Autodesk Inventor part; units mm, degrees
(part 5 of 5)
sketch "Эскиз12" plane through (0, 2, 0) normal (0, 1, 0) x (1, 0, 0)
  line L0 (-0.8, -32.5335) -> (0.8, -32.5335)
  line L1 (0.8, -32.5335) -> (0.8, -39.5335)
  line L2 (0.8, -39.5335) -> (-0.8, -39.5335)
  line L3 (-0.8, -39.5335) -> (-0.8, -32.5335)
  line L4 (-0.8, -32.5335) -> (0.8, -39.5335) construction
  line L5 (35.896, -32.6933) -> (41.3657, -27.2236) construction
  arc A0 (44.1942, -27.2236) -> (41.3657, -27.2236) centre (42.78, -28.6378) ccw construction
  line L6 (44.1942, -27.2236) -> (63.6396, -46.669) construction
  line L7 (63.6396, -46.669) -> (46.669, -63.6396) construction
  line L8 (46.669, -63.6396) -> (27.2236, -44.1942) construction
  arc A1 (27.2236, -41.3657) -> (27.2236, -44.1942) centre (28.6378, -42.78) ccw construction
  line L9 (27.2236, -41.3657) -> (31.4801, -37.1092) construction
  arc A2 (31.4801, -37.1092) -> (35.896, -32.6933) centre (31.9203, -33.1335) ccw construction
  circle A3 centre (0, -54) radius 1.6 construction
  arc A4 (-93.0503, 48.6481) -> (-93.0503, -48.6481) centre (0, 0) ccw construction
  arc A5 (-93.0503, -48.6481) -> (-88.2704, -49.3795) centre (-90.3917, -47.2582) ccw construction
  line L10 (-88.2704, -49.3795) -> (-85.2064, -46.3155) construction
  arc A6 (-73.8927, -46.3155) -> (-85.2064, -46.3155) centre (-79.5495, -51.9723) ccw construction
  line L11 (-73.8927, -46.3155) -> (-46.3155, -73.8927) construction
  arc A7 (-46.3155, -85.2064) -> (-46.3155, -73.8927) centre (-51.9723, -79.5495) ccw construction
  line L12 (-46.3155, -85.2064) -> (-49.3795, -88.2704) construction
  arc A8 (-49.3795, -88.2704) -> (-48.6481, -93.0503) centre (-47.2582, -90.3917) ccw construction
  arc A9 (-48.6481, -93.0503) -> (-45.42, -94.668) centre (0, 0) ccw construction
  arc A10 (-45.42, -94.668) -> (-43.0355, -94.1655) centre (-44.5548, -92.8648) ccw construction
  line L13 (-43.0355, -94.1655) -> (-18.3802, -65.3664) construction
  arc A11 (-17.477, -64.7643) -> (-18.3802, -65.3664) centre (-16.8609, -66.6671) ccw construction
  line L14 (-17.477, -64.7643) -> (-0.6161, -59.3045) construction
  arc A12 (0.6161, -59.3045) -> (-0.6161, -59.3045) centre (0, -61.2072) ccw construction
  line L15 (0.6161, -59.3045) -> (17.477, -64.7643) construction
  arc A13 (18.3802, -65.3664) -> (17.477, -64.7643) centre (16.8609, -66.6671) ccw construction
  line L16 (18.3802, -65.3664) -> (43.0355, -94.1655) construction
  arc A14 (43.0355, -94.1655) -> (45.42, -94.668) centre (44.5548, -92.8648) ccw construction
  arc A15 (45.42, -94.668) -> (48.6481, -93.0503) centre (0, 0) ccw construction
  arc A16 (48.6481, -93.0503) -> (49.3795, -88.2704) centre (47.2582, -90.3917) ccw construction
  line L17 (49.3795, -88.2704) -> (46.3155, -85.2064) construction
  arc A17 (46.3155, -73.8927) -> (46.3155, -85.2064) centre (51.9723, -79.5495) ccw construction
  line L18 (46.3155, -73.8927) -> (73.8927, -46.3155) construction
  arc A18 (85.2064, -46.3155) -> (73.8927, -46.3155) centre (79.5495, -51.9723) ccw construction
  line L19 (85.2064, -46.3155) -> (88.2704, -49.3795) construction
  arc A19 (88.2704, -49.3795) -> (93.0503, -48.6481) centre (90.3917, -47.2582) ccw construction
  arc A20 (93.0503, -48.6481) -> (93.0503, 48.6481) centre (0, 0) ccw construction
  arc A21 (93.0503, 48.6481) -> (88.2704, 49.3795) centre (90.3917, 47.2582) ccw construction
  line L20 (88.2704, 49.3795) -> (85.2064, 46.3155) construction
  arc A22 (73.8927, 46.3155) -> (85.2064, 46.3155) centre (79.5495, 51.9723) ccw construction
  line L21 (73.8927, 46.3155) -> (46.3155, 73.8927) construction
  arc A23 (46.3155, 85.2064) -> (46.3155, 73.8927) centre (51.9723, 79.5495) ccw construction
  line L22 (46.3155, 85.2064) -> (49.3795, 88.2704) construction
  arc A24 (49.3795, 88.2704) -> (48.6481, 93.0503) centre (47.2582, 90.3917) ccw construction
  arc A25 (48.6481, 93.0503) -> (11.8382, 104.3305) centre (0, 0) ccw construction
  arc A26 (11.8382, 104.3305) -> (8.5, 101.3496) centre (11.5, 101.3496) ccw construction
  line L23 (8.5, 101.3496) -> (8.5, 90.5) construction
  arc A27 (7, 89) -> (8.5, 90.5) centre (7, 90.5) ccw construction
  line L24 (7, 89) -> (-7, 89) construction
  arc A28 (-8.5, 90.5) -> (-7, 89) centre (-7, 90.5) ccw construction
  line L25 (-8.5, 90.5) -> (-8.5, 101.3496) construction
  arc A29 (-8.5, 101.3496) -> (-11.8382, 104.3305) centre (-11.5, 101.3496) ccw construction
  arc A30 (-11.8382, 104.3305) -> (-48.6481, 93.0503) centre (0, 0) ccw construction
  arc A31 (-48.6481, 93.0503) -> (-49.3795, 88.2704) centre (-47.2582, 90.3917) ccw construction
  line L26 (-49.3795, 88.2704) -> (-46.3155, 85.2064) construction
  arc A32 (-46.3155, 73.8927) -> (-46.3155, 85.2064) centre (-51.9723, 79.5495) ccw construction
  line L27 (-46.3155, 73.8927) -> (-73.8927, 46.3155) construction
  arc A33 (-85.2064, 46.3155) -> (-73.8927, 46.3155) centre (-79.5495, 51.9723) ccw construction
  line L28 (-85.2064, 46.3155) -> (-88.2704, 49.3795) construction
  arc A34 (-88.2704, 49.3795) -> (-93.0503, 48.6481) centre (-90.3917, 47.2582) ccw construction
  arc A35 (-90.4395, 37.7453) -> (-97.9653, 2.6059) centre (0, 0) ccw construction
  arc A36 (-87.1795, 38.3892) -> (-90.4395, 37.7453) centre (-88.5938, 36.975) ccw construction
  line L29 (-87.1795, 38.3892) -> (-83.085, 34.2947) construction
  arc A37 (-83.085, 34.2947) -> (-76.014, 34.2947) centre (-79.5495, 37.8302) ccw construction
  line L30 (-76.014, 34.2947) -> (-67.8823, 42.4264) construction
  line L31 (-67.8823, 42.4264) -> (-47.1257, 21.6698) construction
  arc A38 (-47.1257, 21.6698) -> (-43.384, 17.9282) centre (-43.1335, 21.9203) ccw construction
  line L32 (-43.384, 17.9282) -> (-26.8701, 1.4142) construction
  arc A39 (-26.8701, -1.4142) -> (-26.8701, 1.4142) centre (-28.2843, 0) ccw construction
  line L33 (-26.8701, -1.4142) -> (-43.384, -17.9282) construction
  arc A40 (-43.384, -17.9282) -> (-47.1257, -21.6698) centre (-43.1335, -21.9203) ccw construction
  line L34 (-47.1257, -21.6698) -> (-67.8823, -42.4264) construction
  line L35 (-67.8823, -42.4264) -> (-76.014, -34.2947) construction
  arc A41 (-76.014, -34.2947) -> (-83.085, -34.2947) centre (-79.5495, -37.8302) ccw construction
  line L36 (-83.085, -34.2947) -> (-87.1795, -38.3892) construction
  arc A42 (-90.4395, -37.7453) -> (-87.1795, -38.3892) centre (-88.5938, -36.975) ccw construction
  arc A43 (-97.9653, -2.6059) -> (-90.4395, -37.7453) centre (0, 0) ccw construction
  arc A44 (-97.9653, -2.6059) -> (-97.9653, 2.6059) centre (-101, 0) ccw construction
  line L37 (29.746, -55.2019) -> (42.4264, -67.8823) construction
  line L38 (42.4264, -67.8823) -> (37.1244, -73.1843) construction
  arc A45 (34.1909, -73.0707) -> (37.1244, -73.1843) centre (35.7102, -71.7701) ccw construction
  line L39 (34.1909, -73.0707) -> (25.4187, -62.8242) construction
  arc A46 (24.842, -61.8893) -> (25.4187, -62.8242) centre (28.1154, -60.5155) ccw construction
  line L40 (24.842, -61.8893) -> (24.3148, -60.6331) construction
  line L41 (24.3148, -60.6331) -> (29.746, -55.2019) construction
  line L42 (-24.3148, -60.6331) -> (-24.842, -61.8893) construction
  arc A47 (-25.4187, -62.8242) -> (-24.842, -61.8893) centre (-28.1154, -60.5155) ccw construction
  line L43 (-25.4187, -62.8242) -> (-34.1909, -73.0707) construction
  arc A48 (-37.1244, -73.1843) -> (-34.1909, -73.0707) centre (-35.7102, -71.7701) ccw construction
  line L44 (-37.1244, -73.1843) -> (-42.4264, -67.8823) construction
  line L45 (-42.4264, -67.8823) -> (-29.746, -55.2019) construction
  line L46 (-29.746, -55.2019) -> (-24.3148, -60.6331) construction
  arc A49 (37.7453, 90.4395) -> (18.0526, 96.3229) centre (0, 0) ccw construction
  arc A50 (38.3892, 87.1795) -> (37.7453, 90.4395) centre (36.975, 88.5938) ccw construction
  line L47 (38.3892, 87.1795) -> (34.2947, 83.085) construction
  arc A51 (34.2947, 83.085) -> (34.2947, 76.014) centre (37.8302, 79.5495) ccw construction
  line L48 (34.2947, 76.014) -> (42.4264, 67.8823) construction
  line L49 (42.4264, 67.8823) -> (21.6698, 47.1257) construction
  arc A52 (21.6698, 47.1257) -> (17.9282, 43.384) centre (21.9203, 43.1335) ccw construction
  line L50 (17.9282, 43.384) -> (1.4142, 26.8701) construction
  arc A53 (-1.4142, 26.8701) -> (1.4142, 26.8701) centre (0, 28.2843) ccw construction
  line L51 (-1.4142, 26.8701) -> (-17.9282, 43.384) construction
  arc A54 (-17.9282, 43.384) -> (-21.6698, 47.1257) centre (-21.9203, 43.1335) ccw construction
  line L52 (-21.6698, 47.1257) -> (-42.4264, 67.8823) construction
  line L53 (-42.4264, 67.8823) -> (-34.2947, 76.014) construction
  arc A55 (-34.2947, 76.014) -> (-34.2947, 83.085) centre (-37.8302, 79.5495) ccw construction
  line L54 (-34.2947, 83.085) -> (-38.3892, 87.1795) construction
  arc A56 (-37.7453, 90.4395) -> (-38.3892, 87.1795) centre (-36.975, 88.5938) ccw construction
  arc A57 (-18.0526, 96.3229) -> (-37.7453, 90.4395) centre (0, 0) ccw construction
  arc A58 (-14.5, 93.3742) -> (-18.0526, 96.3229) centre (-17.5, 93.3742) ccw construction
  line L55 (-14.5, 93.3742) -> (-14.5, 87) construction
  arc A59 (-14.5, 87) -> (-11.5, 84) centre (-11.5, 87) ccw construction
  line L56 (-11.5, 84) -> (11.5, 84) construction
  arc A60 (11.5, 84) -> (14.5, 87) centre (11.5, 87) ccw construction
  line L57 (14.5, 87) -> (14.5, 93.3742) construction
  arc A61 (18.0526, 96.3229) -> (14.5, 93.3742) centre (17.5, 93.3742) ccw construction
  line L58 (-11.01, -20.1936) -> (-11.01, -27.9806) construction
  line L59 (-11.01, -27.9806) -> (-13.3848, -30.3553) construction
  line L60 (-19.0416, -30.3553) -> (-13.3848, -30.3553) construction
  line L61 (-19.0416, -30.3553) -> (-20.5061, -28.8909) construction
  arc A62 (-20.5061, -28.8909) -> (-21.9203, -28.3051) centre (-21.9203, -30.3051) ccw construction
  line L62 (-21.9203, -28.3051) -> (-33.2132, -28.3051) construction
  line L63 (-33.2132, -28.3051) -> (-37.8302, -23.6881) construction
  arc A63 (-37.8302, -20.8597) -> (-37.8302, -23.6881) centre (-36.416, -22.2739) ccw construction
  line L64 (-37.8302, -20.8597) -> (-24.6871, -7.7166) construction
  arc A64 (-21.4111, -8.4003) -> (-24.6871, -7.7166) centre (-23.2729, -9.1308) ccw construction
  arc A65 (-21.4111, -8.4003) -> (-11.01, -20.1936) centre (0, 0) ccw construction
  circle A66 centre (-37.8302, -79.5495) radius 1.6 construction
  circle A67 centre (37.8302, -79.5495) radius 1.6 construction
  circle A68 centre (20.5578, -60.8546) radius 1.55 construction
  circle A69 centre (-20.5578, -60.8546) radius 1.55 construction
  circle A70 centre (79.5495, 37.8302) radius 1.6 construction
  circle A71 centre (37.8302, 79.5495) radius 1.6 construction
  circle A72 centre (79.5495, -37.8302) radius 1.6 construction
  circle A73 centre (-79.5495, -37.8302) radius 1.6 construction
  circle A74 centre (-79.5495, 37.8302) radius 1.6 construction
  circle A75 centre (-37.8302, 79.5495) radius 1.6 construction
  circle A76 centre (22, 0) radius 1.6 construction
  circle A77 centre (0, -22) radius 1.6 construction
  circle A78 centre (-22, 0) radius 1.6 construction
  circle A79 centre (0, 22) radius 1.6 construction
  circle A80 centre (43.1335, -21.9203) radius 1.6 construction
  circle A81 centre (0, 0) radius 18 construction
  circle A82 centre (-43.1335, 21.9203) radius 1.6 construction
  circle A83 centre (-21.9203, -43.1335) radius 1.6 construction
  circle A84 centre (21.9203, 43.1335) radius 1.6 construction
  circle A85 centre (43.1335, 21.9203) radius 1.6 construction
  circle A86 centre (-43.1335, -21.9203) radius 1.6 construction
  circle A87 centre (21.9203, -43.1335) radius 1.6 construction
  line L65 (37.8302, 20.8597) -> (24.6871, 7.7166) construction
  arc A88 (21.4111, 8.4003) -> (24.6871, 7.7166) centre (23.2729, 9.1308) ccw construction
  arc A89 (21.4111, 8.4003) -> (8.4003, 21.4111) centre (0, 0) ccw construction
  arc A90 (7.7166, 24.6871) -> (8.4003, 21.4111) centre (9.1308, 23.2729) ccw construction
  line L66 (7.7166, 24.6871) -> (20.8597, 37.8302) construction
  arc A91 (23.6881, 37.8302) -> (20.8597, 37.8302) centre (22.2739, 36.416) ccw construction
  line L67 (23.6881, 37.8302) -> (37.8302, 23.6881) construction
  arc A92 (37.8302, 20.8597) -> (37.8302, 23.6881) centre (36.416, 22.2739) ccw construction
  arc A93 (-24.6871, 7.7166) -> (-21.4111, 8.4003) centre (-23.2729, 9.1308) ccw construction
  line L68 (-24.6871, 7.7166) -> (-37.8302, 20.8597) construction
  arc A94 (-37.8302, 23.6881) -> (-37.8302, 20.8597) centre (-36.416, 22.2739) ccw construction
  line L69 (-37.8302, 23.6881) -> (-23.6881, 37.8302) construction
  arc A95 (-20.8597, 37.8302) -> (-23.6881, 37.8302) centre (-22.2739, 36.416) ccw construction
  line L70 (-20.8597, 37.8302) -> (-7.7166, 24.6871) construction
  arc A96 (-8.4003, 21.4111) -> (-7.7166, 24.6871) centre (-9.1308, 23.2729) ccw construction
  arc A97 (-8.4003, 21.4111) -> (-21.4111, 8.4003) centre (0, 0) ccw construction
  circle A98 centre (-21.9203, 43.1335) radius 1.6 construction
  line L71 (-46.669, 63.6396) -> (-27.2236, 44.1942) construction
  arc A99 (-27.2236, 41.3657) -> (-27.2236, 44.1942) centre (-28.6378, 42.78) ccw construction
  line L72 (-27.2236, 41.3657) -> (-41.3657, 27.2236) construction
  arc A100 (-44.1942, 27.2236) -> (-41.3657, 27.2236) centre (-42.78, 28.6378) ccw construction
  line L73 (-44.1942, 27.2236) -> (-63.6396, 46.669) construction
  line L74 (-63.6396, 46.669) -> (-46.669, 63.6396) construction
  line L75 (63.6396, 46.669) -> (44.1942, 27.2236) construction
  arc A101 (41.3657, 27.2236) -> (44.1942, 27.2236) centre (42.78, 28.6378) ccw construction
  line L76 (41.3657, 27.2236) -> (27.2236, 41.3657) construction
  arc A102 (27.2236, 44.1942) -> (27.2236, 41.3657) centre (28.6378, 42.78) ccw construction
  line L77 (27.2236, 44.1942) -> (46.669, 63.6396) construction
  line L78 (46.669, 63.6396) -> (63.6396, 46.669) construction
  line L79 (-10.11, -40.3943) -> (-10.11, -55.0209) construction
  line L80 (-10.11, -55.0209) -> (-14.5119, -56.4463) construction
  arc A103 (-15.1585, -56.5907) -> (-14.5119, -56.4463) centre (-15.6055, -53.069) ccw construction
  line L81 (-15.1585, -56.5907) -> (-17.9282, -56.9423) construction
  line L82 (-17.9282, -56.9423) -> (-17.9282, -43.384) construction
  line L83 (-17.9282, -43.384) -> (-13.5242, -38.9801) construction
  arc A104 (-10.11, -40.3943) -> (-13.5242, -38.9801) centre (-12.11, -40.3943) ccw construction
  arc A105 (90.4395, -37.7453) -> (97.9653, -2.6059) centre (0, 0) ccw construction
  arc A106 (87.1795, -38.3892) -> (90.4395, -37.7453) centre (88.5938, -36.975) ccw construction
  line L84 (87.1795, -38.3892) -> (83.085, -34.2947) construction
  arc A107 (83.085, -34.2947) -> (76.014, -34.2947) centre (79.5495, -37.8302) ccw construction
  line L85 (76.014, -34.2947) -> (67.8823, -42.4264) construction
  line L86 (67.8823, -42.4264) -> (47.1257, -21.6698) construction
  arc A108 (47.1257, -21.6698) -> (43.384, -17.9282) centre (43.1335, -21.9203) ccw construction
  line L87 (43.384, -17.9282) -> (26.8701, -1.4142) construction
  arc A109 (26.8701, 1.4142) -> (26.8701, -1.4142) centre (28.2843, 0) ccw construction
  line L88 (26.8701, 1.4142) -> (43.384, 17.9282) construction
  arc A110 (43.384, 17.9282) -> (47.1257, 21.6698) centre (43.1335, 21.9203) ccw construction
  line L89 (47.1257, 21.6698) -> (67.8823, 42.4264) construction
  line L90 (67.8823, 42.4264) -> (76.014, 34.2947) construction
  arc A111 (76.014, 34.2947) -> (83.085, 34.2947) centre (79.5495, 37.8302) ccw construction
  line L91 (83.085, 34.2947) -> (87.1795, 38.3892) construction
  arc A112 (90.4395, 37.7453) -> (87.1795, 38.3892) centre (88.5938, 36.975) ccw construction
  arc A113 (97.9653, 2.6059) -> (90.4395, 37.7453) centre (0, 0) ccw construction
  arc A114 (97.9653, 2.6059) -> (97.9653, -2.6059) centre (101, 0) ccw construction
  circle A115 centre (-101, 0) radius 1.6 construction
  circle A116 centre (101, 0) radius 1.6 construction
  circle A117 centre (90.3659, 45.1111) radius 1.6 construction
  circle A118 centre (-90.3659, -45.1111) radius 1.6 construction
  circle A119 centre (45.1111, 90.3659) radius 1.6 construction
  circle A120 centre (-45.1111, -90.3659) radius 1.6 construction
  circle A121 centre (90.3659, -45.1111) radius 1.6 construction
  circle A122 centre (-90.3659, 45.1111) radius 1.6 construction
  circle A123 centre (-45.1111, 90.3659) radius 1.6 construction
  circle A124 centre (45.1111, -90.3659) radius 1.6 construction
  line L92 (-31.4801, -37.1092) -> (-27.2236, -41.3657) construction
  arc A125 (-27.2236, -44.1942) -> (-27.2236, -41.3657) centre (-28.6378, -42.78) ccw construction
  line L93 (-27.2236, -44.1942) -> (-46.669, -63.6396) construction
  line L94 (-46.669, -63.6396) -> (-63.6396, -46.669) construction
  line L95 (-63.6396, -46.669) -> (-44.1942, -27.2236) construction
  arc A126 (-41.3657, -27.2236) -> (-44.1942, -27.2236) centre (-42.78, -28.6378) ccw construction
  line L96 (-41.3657, -27.2236) -> (-35.896, -32.6933) construction
  arc A127 (-35.896, -32.6933) -> (-31.4801, -37.1092) centre (-31.9203, -33.1335) ccw construction
  line L97 (13.3848, -30.3553) -> (7.7166, -24.6871) construction
  arc A128 (8.4003, -21.4111) -> (7.7166, -24.6871) centre (9.1308, -23.2729) ccw construction
  arc A129 (8.4003, -21.4111) -> (21.4111, -8.4003) centre (0, 0) ccw construction
  arc A130 (24.6871, -7.7166) -> (21.4111, -8.4003) centre (23.2729, -9.1308) ccw construction
  line L98 (24.6871, -7.7166) -> (37.8302, -20.8597) construction
  arc A131 (37.8302, -23.6881) -> (37.8302, -20.8597) centre (36.416, -22.2739) ccw construction
  line L99 (37.8302, -23.6881) -> (33.2132, -28.3051) construction
  line L100 (33.2132, -28.3051) -> (21.9203, -28.3051) construction
  arc A132 (21.9203, -28.3051) -> (20.5061, -28.8909) centre (21.9203, -30.3051) ccw construction
  line L101 (20.5061, -28.8909) -> (19.0416, -30.3553) construction
  line L102 (13.3848, -30.3553) -> (19.0416, -30.3553) construction
  circle A133 centre (-21.9203, -33.1335) radius 1.6 construction
  circle A134 centre (21.9203, -33.1335) radius 1.6 construction
  circle A135 centre (-31.9203, -33.1335) radius 1.6 construction
  circle A136 centre (31.9203, -33.1335) radius 1.6 construction
  circle A137 centre (-7.01, -24.698) radius 1.75 construction
  circle A138 centre (7.01, -46.7128) radius 1.75 construction
  line L103 (13.5242, -38.9801) -> (17.9282, -43.384) construction
  line L104 (17.9282, -43.384) -> (17.9282, -56.9423) construction
  line L105 (17.9282, -56.9423) -> (15.1585, -56.5907) construction
  arc A139 (14.5119, -56.4463) -> (15.1585, -56.5907) centre (15.6055, -53.069) ccw construction
  line L106 (14.5119, -56.4463) -> (10.11, -55.0209) construction
  line L107 (10.11, -55.0209) -> (10.11, -40.3943) construction
  arc A140 (13.5242, -38.9801) -> (10.11, -40.3943) centre (12.11, -40.3943) ccw construction
  line L108 (0, -22) -> (0, -54) construction
  line L109 (-3.4311, -34.9763) -> (-2.6311, -33.5907)
  line L110 (-2.6311, -33.5907) -> (3.4311, -37.0907)
  line L111 (2.6311, -38.4763) -> (-3.4311, -34.9763)
  line L112 (3.4311, -37.0907) -> (2.6311, -38.4763)
  line L113 (-2.6311, -38.4763) -> (-3.4311, -37.0907)
  line L114 (-3.4311, -37.0907) -> (2.6311, -33.5907)
  line L115 (3.4311, -34.9763) -> (-2.6311, -38.4763)
  line L116 (2.6311, -33.5907) -> (3.4311, -34.9763)
  line L117 (0.8, -39.5335) -> (-0.8, -39.5335)
  line L118 (-0.8, -39.5335) -> (-0.8, -32.5335)
  line L119 (0.8, -32.5335) -> (0.8, -39.5335)
  line L120 (-0.8, -32.5335) -> (0.8, -32.5335)
  line L121 (3.4311, -37.0907) -> (2.6311, -38.4763)
  line L122 (2.6311, -38.4763) -> (-3.4311, -34.9763)
  line L123 (-2.6311, -33.5907) -> (3.4311, -37.0907)
  line L124 (-3.4311, -34.9763) -> (-2.6311, -33.5907)
  line L125 (2.6311, -33.5907) -> (3.4311, -34.9763)
  line L126 (3.4311, -34.9763) -> (-2.6311, -38.4763)
  line L127 (-3.4311, -37.0907) -> (2.6311, -33.5907)
  line L128 (-2.6311, -38.4763) -> (-3.4311, -37.0907)
  point P0 (0, -36.0335)
  point P1 (0.8, -37.4192)
  point P2 (1.6, -36.0335)
  point P3 (0.8, -34.6479)
  point P4 (-0.8, -34.6479)
  point P5 (-1.6, -36.0335)
  point P6 (-0.8, -37.4192)
  dimension "d162" = 1.6
  dimension "d163" = 7
  dimension "d166" = 360
  constraints: 52 end point, 2 parallel, 1 horizontal, 1 midpoint, 1 perpendicular, 1 point on line, 1 vertical, 50 other
  measures "d162" distance of L1.end L2.end
  measures "d163" distance of L0.end L1.end
extrude "Выдавливание15" [suppressed]
fillet "Сопряжение2" [suppressed]
